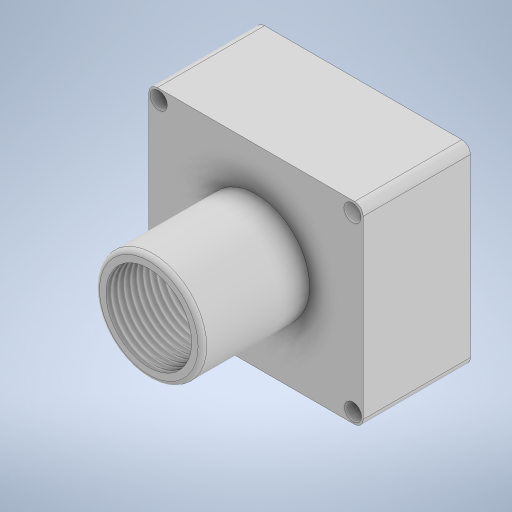
# Autodesk Inventor part: PIEZA PRÁCTICA NO.1
Saved by Autodesk Inventor 2024 (Build 280153000, 153)
## iProperties
Created: 2024-02-16
Part Number: PIEZA PRÁCTICA NO.1
Material: Genérico
Document SubType Name: Modeling
Designer: carlo
Density: 1 g/cm^3
Appearance: Valor por defecto
Author: carlo
Autodesk Inventor part; units mm, degrees
ref_plane "YZ Plane" through (0, 0, 0) normal (1, 0, 0) x (0, 1, 0)
ref_plane "XZ Plane" through (0, 0, 0) normal (0, 1, 0) x (-1, 0, 0)
ref_plane "XY Plane" through (0, 0, 0) normal (0, 0, 1) x (1, 0, 0)
sketch "Boceto1" plane through (0, 0, 0) normal (0, 0, 1) x (1, 0, 0)
  line L0 (-46, -45) -> (46, -45)
  line L1 (50, -41) -> (50, 41)
  line L2 (46, 45) -> (-46, 45)
  line L3 (-50, 41) -> (-50, -41)
  line L4 (-50, -45) -> (50, 45) construction
  line L5 (50, -45) -> (-50, 45) construction
  arc A0 (-46, 45) -> (-50, 41) centre (-46, 41) ccw
  arc A1 (50, 41) -> (46, 45) centre (46, 41) ccw
  arc A2 (-50, -41) -> (-46, -45) centre (-46, -41) ccw
  arc A3 (46, -45) -> (50, -41) centre (46, -41) ccw
  circle A4 centre (45, 40) radius 4
  line L6 (-46, 41) -> (-45.331, 40.2567)
  circle A5 centre (-45.3262, 40.2313) radius 4
  line L7 (46, -41) -> (45.2567, -40.331)
  circle A6 centre (45.2538, -40.3293) radius 4
  circle A7 centre (-45.2619, -40.3231) radius 4
  point P0 (0, 0)
  dimension "d0" = 100
  dimension "d1" = 90
  dimension "d50" = 1
  dimension "d51" = 1
  constraints: 16 end point, 8 centre point, 8 point on circle, 3 parallel, 2 midpoint, 1 horizontal, 1 perpendicular
  measures "d0" distance of L5.end L4.end
  measures "d1" distance of L4.end L5.start
  measures "d50" distance of L6.start L6.end
  measures "d51" distance of L7.start L7.end
extrude "Extrusión1" add sketch "Boceto1" along normal blind 50
sketch "Boceto2" plane through (0, 0, 50) normal (0, 0, 1) x (1, 0, 0)
  circle A0 centre (0, 0) radius 25
  dimension "d4" = 50
  constraints: 1 centre point, 1 coincident
  measures "d4" diameter of A0
extrude "Extrusión2" add sketch "Boceto2" along normal blind 50
sketch "Boceto3" plane through (0, 0, 100) normal (0, 0, 1) x (1, 0, 0)
  circle A0 centre (0, 0) radius 20
  dimension "d7" = 40
  constraints: 1 centre point, 1 coincident
  measures "d7" diameter of A0
extrude "Extrusión3" cut sketch "Boceto3" against normal blind 30
sketch "Boceto4" plane through (0, 0, 50) normal (0, 0, 1) x (1, 0, 0)
  point P0 (0, 0)
fillet "Empalme1" radius 2 1 edges at (-25, 0, 100)
sketch "Boceto7" plane through (0, 0, 50) normal (0, 0, 1) x (1, 0, 0)
  point P0 (0, 0)
thread "Rosca1" size "M40x3" class "6H" standard "ANSI Metric M Profile" full length
